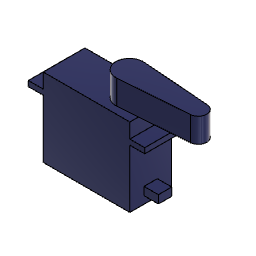
Hexapod Leg v4 (Autodesk Fusion 360 archive; units mm, degrees)
design "smaller servo"
Autodesk Fusion 360 part; units mm, degrees
sketch "Sketch3" plane through (0, 0, 0) normal (0, 1, 0) x (1, 0, 0)
  line L0 (0, 0) -> (40.9, 0)
  line L1 (40.9, 0) -> (40.9, -37)
  line L2 (40.9, -37) -> (0, -37)
  line L3 (0, -37) -> (0, 0)
  line L4 (-7.05, -30) -> (47.95, -30)
  line L5 (47.95, -30) -> (47.95, -27.5)
  line L6 (47.95, -27.5) -> (-7.05, -27.5)
  line L7 (-7.05, -27.5) -> (-7.05, -30)
  line L8 (20.45, 0) -> (20.45, -37) construction
  dimension "d8" = 40.9
  dimension "d9" = 37
  dimension "d10" = 2.5
  dimension "d11" = 27.5
  dimension "d12" = 55
  dimension "d13" = 27.5
  constraint horizontal L0
  constraint vertical L1
  constraint horizontal L2
  constraint vertical L3
  constraint coincident L0.start L3.end
  constraint horizontal L4
  constraint perpendicular L4 L5
  constraint perpendicular L5 L6
  constraint perpendicular L4 L7
  constraint midpoint L0 L8.start
  constraint midpoint L2 L8.end
  measures "d8" distance of L0.start L0.end
  measures "d9" distance of L0.start L2.end
  measures "d10" distance of L4.end L5.end
  measures "d11" distance of L0 L6
  measures "d12" distance of L4.start L4.end
  measures "d13" distance of L5 L8
extrude "Extrude2" add sketch "Sketch3" along normal blind 19.7 makes body 1
sketch "Sketch4" plane through (40.9, 0, 0) normal (1, 0, 0) x (0, 1, 0)
  line L0 (0, 27.5) -> (0, 0) construction
  line L1 (0, 0) -> (19.7, 0)
  line L2 (19.7, 0) -> (19.7, 27.5)
  line L3 (19.7, 27.5) -> (0, 27.5)
  line L4 (6.7, 7.3) -> (13, 7.3)
  line L5 (13, 7.3) -> (13, 3.5)
  line L6 (13, 3.5) -> (6.7, 3.5)
  line L7 (6.7, 3.5) -> (6.7, 7.3)
  line L8 (9.85, 0) -> (9.85, 21.995) construction
  dimension "d16" = 6.3
  dimension "d17" = 3.8
  dimension "d18" = 3.5
  dimension "d19" = 3.15
  constraint horizontal L4
  constraint vertical L5
  constraint horizontal L6
  constraint vertical L7
  constraint midpoint L1 L8.start
  constraint perpendicular L1 L8
  measures "d16" distance of L4.start L4.end
  measures "d17" distance of L4.end L5.end
  measures "d18" distance of L1 L6
  measures "d19" distance of L5 L8
extrude "Extrude3" add sketch "Sketch4" along normal blind 6.8 bodies 1
sketch "Sketch5" plane through (0, 0, 37) normal (0, 0, 1) x (-1, 0, 0)
  line L0 (0, 0) -> (-40.9, 0)
  line L1 (-40.9, 0) -> (-40.9, -19.7)
  line L2 (-40.9, -19.7) -> (0, -19.7)
  line L3 (0, -19.7) -> (0, 0)
  line L4 (-40.9, -9.85) -> (-22.3906, -9.85) construction
  circle A0 centre (-30.9, -9.85) radius 6.5
  line L5 (-30.9, -9.85) -> (-63.4, -9.85) construction
  circle A1 centre (-63.4, -9.85) radius 4
  line L6 (-30.9, -9.85) -> (-30.9, -16.35) construction
  line L7 (-30.9, -16.35) -> (-63.7054, -13.8383)
  line L8 (-31.4, -3.3693) -> (-63.7077, -5.8619)
  dimension "d27" = 13
  dimension "d28" = 10
  dimension "d29" = 32.5
  dimension "d30" = 8
  constraint midpoint L1 L4.start
  constraint perpendicular L1 L4
  constraint coincident L4 A0.centre
  constraint coincident A0.centre L5.start
  constraint parallel L4 L5
  constraint coincident L5.end A1.centre
  constraint coincident A0 L6.end
  constraint perpendicular L5 L6
  constraint coincident A1 L7.end
  constraint tangent A1 L7
  constraint coincident A0 L8.start
  constraint coincident A1 L8.end
  constraint tangent A1 L8
  constraint tangent A0 L8
  measures "d27" diameter of A0
  measures "d28" distance of L1 A0.centre
  measures "d29" distance of A0.centre L5.end
  measures "d30" diameter of A1
extrude "Extrude1" add sketch "Sketch5" along normal blind 11.5 separate body contours L1 A0 L7 L8 | L1 A1 L7 L8 | A0 L7 | A1 picked at (-31.6893, -8.3697) makes body 2 in component "Component"
component "Component" placed x (1, 0, 0) y (0, 1, 0) z (0, 0, 1) at (0, 0, 0)
